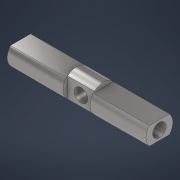
# Autodesk Inventor part: Z25_Slide_Spacer
Saved by Autodesk Inventor 2022 (Build 260153000, 153)
## iProperties
Created: 2023-02-13
Part Number: Z25_Slide_Spacer
Material: Stainless Steel
Document SubType Name: Modeling
Designer: dzw04
Density: 8 g/cm^3
Appearance: Semi-Polished
Author: dzw04
Autodesk Inventor part; units mm, degrees
ref_plane "YZ Plane" through (0, 0, 0) normal (1, 0, 0) x (0, 1, 0)
ref_plane "XZ Plane" through (0, 0, 0) normal (0, 1, 0) x (-1, 0, 0)
ref_plane "XY Plane" through (0, 0, 0) normal (0, 0, 1) x (1, 0, 0)
sketch "Sketch1" plane through (0, 0, 0) normal (1, 0, 0) x (0, 1, 0)
  circle A0 centre (0, 0) radius 3
  dimension "d0" = 6
  constraints: 1 centre point, 1 coincident
  measures "d0" diameter of A0
extrude "Extrusion1" add sketch "Sketch1" along normal mid plane 31
sketch "Sketch2" plane through (0, 0, 0) normal (1, 0, 0) x (0, 1, 0)
  circle A0 centre (0, 0) radius 3 projected
  line L0 (0, 3) -> (0, 2)
  line L1 (-3.5, 2) -> (3.5, 2)
  line L2 (3.5, 2) -> (3.5, 3)
  line L3 (3.5, 3) -> (-3.5, 3)
  line L4 (-3.5, 3) -> (-3.5, 2)
  line L5 (-3.5, 2) -> (3.5, 3) construction
  line L6 (3.5, 2) -> (-3.5, 3) construction
  point P0 (0, 2.5)
  dimension "d3" = 1
  dimension "d4" = 7
  dimension "d5" = 1
  constraints: 14 end point, 3 midpoint, 2 parallel, 1 horizontal, 1 perpendicular, 1 vertical, 1 vertical alignment, 1 other
  measures "d3" distance of L0.start L0.end
  measures "d4" distance of L3.end L2.end
  measures "d5" distance of L2.end L1.end
extrude "Extrusion2" cut sketch "Sketch2" along normal mid plane 6 contours L1 L0 A0 | A0 L3 L2 L1 | L1 L4 L3 A0 | A0 L0 L1
sketch "Sketch3" plane through (-3, 2.2361, 2) normal (0, 0, 1) x (1, 0, 0)
  circle A0 centre (3, -2.2361) radius 1.5
  dimension "d8" = 3
  constraints: 1 centre point, 1 coincident
  measures "d8" diameter of A0
extrude "Extrusion3" cut sketch "Sketch3" against normal through all
sketch "Sketch4" plane through (15.5, 0, 0) normal (1, 0, 0) x (0, 0, -1)
  circle A0 centre (0, 0) radius 1.5
  circle A1 centre (0, 0) radius 3
  line L0 (-3, -2) -> (3, -2)
  line L1 (3, -2) -> (3, 2)
  line L2 (3, 2) -> (-3, 2)
  line L3 (-3, 2) -> (-3, -2)
  line L4 (-3, -2) -> (3, 2) construction
  line L5 (3, -2) -> (-3, 2) construction
  point P0 (2.2361, -2)
  point P1 (-2.2361, -2)
  point P2 (-2.2361, 2)
  point P3 (2.2361, 2)
  dimension "d11" = 3
  dimension "d12" = 6
  dimension "d13" = 6
  dimension "d14" = 4
  constraints: 12 end point, 2 centre point, 2 coincident, 2 midpoint, 2 parallel, 1 horizontal, 1 perpendicular
  measures "d11" diameter of A0
  measures "d12" diameter of A1
  measures "d13" distance of L2.end L1.end
  measures "d14" distance of L1.end L0.end
extrude "Extrusion4" cut sketch "Sketch4" against normal blind 5.5 contours A0 | L2 A1 | A1 L0
sketch "Sketch5" plane through (-15.5, 0, 0) normal (-1, 0, 0) x (0, 0, 1)
  circle A0 centre (0, 0) radius 1.5 projected
  line L0 (2.2361, -2) -> (-2.2361, -2) projected
  arc A1 (-2.2361, 2) -> (-2.2361, -2) centre (0, 0) ccw projected
  line L1 (-2.2361, 2) -> (2.2361, 2) projected
  arc A2 (2.2361, -2) -> (2.2361, 2) centre (0, 0) ccw projected
  circle A3 centre (0, 0) radius 3
  dimension "d17" = 6
  constraints: 1 centre point, 1 coincident
  measures "d17" diameter of A3
extrude "Extrusion5" cut sketch "Sketch5" against normal blind 5.5 contours A0 | A3 L0 | A3 L1
move faces "Move1" translate (7, 0, 0) faces at (-10, 2.3333, 0)
move faces "Move2" translate (-7, 0, 0) faces at (10, 2.1409, 0.5898) (13.6667, 2, 0.7454)
body "Solid1"
